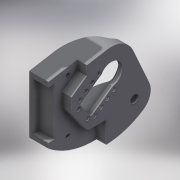
# Autodesk Inventor part: Arm - right shoulder v3
Saved by Autodesk Inventor 2017 (Build 210142000, 142)
## iProperties
Created: 2016-08-10
Part Number: Arm - right shoulder v3
Material: Generic
Document SubType Name: Modeling
Designer: Ali
Density: 1 g/cm^3
Appearance: Default
Author: Ali
Autodesk Inventor part; units mm, degrees
ref_plane "YZ Plane" through (0, 0, 0) normal (1, 0, 0) x (0, 1, 0)
ref_plane "XZ Plane" through (0, 0, 0) normal (0, 1, 0) x (-1, 0, 0)
ref_plane "XY Plane" through (0, 0, 0) normal (0, 0, 1) x (1, 0, 0)
sketch "Sketch1" plane through (0, 0, 0) normal (1, 0, 0) x (0, 1, 0)
  line L0 (0, 30) -> (51.1353, 38.6498)
  line L1 (78.1197, 24.2221) -> (94.819, -13.049)
  line L2 (0, -30) -> (0, 30)
  arc A0 (78.1197, 24.2221) -> (51.1353, 38.6498) centre (55.305, 14) ccw
  arc A1 (88.6362, -34.2101) -> (94.819, -13.049) centre (79.305, -20) ccw
  arc A2 (0, -30) -> (88.6362, -34.2101) centre (47.2144, 28.8695) ccw
  point P0 (0, 0)
  dimension "d14" = 55.305
  dimension "d15" = 14
  dimension "d16" = 17
  dimension "d17" = 34
  dimension "d18" = 24
  dimension "d19" = 25
  dimension "d25" = 60
  dimension "d26" = 30
  constraints: 7 end point, 6 point on circle, 4 tangent, 3 centre point, 1 midpoint, 1 vertical
  measures "d14" horizontal distance of point (0, 0) A0.centre
  measures "d15" vertical distance of point (0, 0) A0.centre
  measures "d16" radius of A1
  measures "d17" vertical distance of A1.centre A0.centre
  measures "d18" horizontal distance of A1.centre A0.centre
  measures "d19" radius of A0
  measures "d25" distance of L2.start L0.start
  measures "d26" distance of L0.start point (0, 0)
extrude "Extrusion1" add sketch "Sketch1" along normal blind 30
sketch "Sketch2" plane through (30, 0, 0) normal (1, 0, 0) x (0, 0, -1)
  circle A0 centre (-14, 55.305) radius 11.4
  arc A1 (-24.2221, 78.1197) -> (-38.6498, 51.1353) centre (-14, 55.305) ccw projected
  line L0 (-14, 55.305) -> (7.0104, 55.305) construction
  line L1 (-14, 55.305) -> (-0.1357, 35.6656) construction
  line L2 (-22.3737, 49.3936) -> (-3.342, 22.4345)
  line L3 (-3.342, 22.4345) -> (5.0317, 28.3459)
  line L4 (13.4054, 34.2572) -> (-5.6263, 61.2164)
  line L5 (-5.6263, 61.2164) -> (-22.3737, 49.3936)
  line L6 (5.0317, 28.3459) -> (13.4054, 34.2572)
  point P0 (0, 0)
  dimension "d6" = 22.8
  dimension "d8" = 54.78
  dimension "d9" = 20.5
  dimension "d10" = 33
  constraints: 14 end point, 6 perpendicular, 1 centre point, 1 coincident, 1 collinear, 1 horizontal, 1 midpoint, 1 point on line
  measures "d6" diameter of A0
  measures "d8" angle of L1 L0
  measures "d9" distance between parallel lines of L4 L2
  measures "d10" distance between parallel lines of L5 L3
extrude "Extrusion2" cut sketch "Sketch2" against normal through all
sketch "Sketch3" plane through (0, 0, 0) normal (-1, 0, 0) x (0, 0, 1)
  line L0 (19.496, 45.3173) -> (3.342, 22.4345) projected
  line L1 (3.342, 22.4345) -> (-13.4054, 34.2572) projected
  line L2 (-13.4054, 34.2572) -> (2.7487, 57.14) projected
  arc A0 (19.496, 45.3173) -> (2.7487, 57.14) centre (14, 55.305) ccw projected
  line L3 (30, 0) -> (38.6498, 51.1353) projected
  arc A1 (38.6498, 51.1353) -> (24.2221, 78.1197) centre (14, 55.305) ccw projected
  line L4 (24.2221, 78.1197) -> (-13.049, 94.819) projected
  arc A2 (-13.049, 94.819) -> (-34.2101, 88.6362) centre (-20, 79.305) ccw projected
  line L5 (-30, 0) -> (30, 0) projected
  line L6 (0.7237, 65.6142) -> (-22.5217, 32.6862)
  line L7 (2.7487, 57.14) -> (-13.4054, 34.2572) projected
  line L8 (-22.5217, 32.6862) -> (4.9137, 13.3183)
  line L9 (4.9137, 13.3183) -> (27.7177, 45.621)
  arc A3 (-2.0441, 50.3509) -> (14.7033, 38.5282) centre (14, 55.305) ccw construction
  arc A4 (0.2823, 64.989) -> (-2.0441, 50.3509) centre (14, 55.305) ccw construction
  arc A5 (27.7177, 45.621) -> (0.2823, 64.989) centre (14, 55.305) ccw
  arc A6 (14.7033, 38.5282) -> (27.7177, 45.621) centre (14, 55.305) ccw construction
  arc A7 (-34.2101, 88.6362) -> (-30, 0) centre (28.8695, 47.2144) ccw projected
  point P0 (0, 0)
  dimension "d20" = 33.583
  dimension "d21" = 16.7915
  dimension "d22" = 39.541
  constraints: 8 point on circle, 6 end point, 4 centre point, 3 point on line, 2 parallel, 2 tangent, 1 coincident, 1 perpendicular
  measures "d20" distance of L6.end L8.end
  measures "d21" distance from line of A0.centre L9
  measures "d22" distance from line of L8 A0.centre
extrude "Extrusion3" cut sketch "Sketch3" against normal blind 26 contours A5 L9 L8 L6
sketch "Sketch4" plane through (0, 0, 0) normal (-1, 0, 0) x (0, 0, 1)
  arc A0 (-13.049, 94.819) -> (-34.2101, 88.6362) centre (-20, 79.305) ccw projected
  arc A1 (-20, 62.305) -> (-3.8668, 84.6641) centre (-20, 79.305) ccw
  line L0 (-20, 62.305) -> (-49.8582, 62.305)
  line L1 (-49.8582, 62.305) -> (-49.8582, 92.5555)
  line L2 (-49.8582, 92.5555) -> (-2.7738, 107.9881)
  arc A2 (-3.8668, 84.6641) -> (-20, 62.305) centre (-20, 79.305) ccw construction
  line L3 (-20, 79.305) -> (-20, 114.7318) construction
  line L4 (2.7487, 57.14) -> (-13.4054, 34.2572) projected
  line L5 (-13.4054, 34.2572) -> (3.342, 22.4345) projected
  arc A3 (19.496, 45.3173) -> (2.7487, 57.14) centre (14, 55.305) ccw projected
  line L6 (-13.049, 94.819) -> (24.2221, 78.1197) projected
  line L7 (24.2221, 78.1197) -> (18.4359, 107.9881)
  line L8 (18.4359, 107.9881) -> (-2.7738, 107.9881)
  line L9 (24.2221, 78.1197) -> (-13.049, 94.819) projected
  arc A4 (0.6004, 88.7034) -> (-3.8668, 84.6641) centre (-0.7447, 85.7011) ccw
  point P0 (0, 0)
  dimension "d29" = 17
  constraints: 12 end point, 7 point on circle, 3 centre point, 3 tangent, 2 horizontal, 1 coincident, 1 perpendicular, 1 point on line, 1 vertical
  measures "d29" radius of A2
extrude "Extrusion4" cut sketch "Sketch4" against normal blind 24
sketch "Sketch5" plane through (0, 0, 0) normal (0, 0, 1) x (1, 0, 0)
  arc A0 (21, 63.7233) -> (0, 26.742) centre (43.0624, 26.742) ccw
  line L0 (0, 26.742) -> (0, 0)
  line L1 (34.277, 106.8627) -> (34.277, 0)
  line L2 (34.277, 0) -> (0, 0)
  line L3 (24, 94.819) -> (24, 88.7034) projected
  line L4 (21, 106.8627) -> (21, 63.7233)
  line L5 (21, 106.8627) -> (34.277, 106.8627)
  point P0 (24, 78.1197)
  dimension "d81" = 3
  constraints: 10 end point, 3 vertical, 2 point on circle, 1 centre point, 1 coincident, 1 horizontal, 1 perpendicular, 1 tangent
  measures "d81" distance between parallel lines of L3 L4
extrude "Extrusion5" cut sketch "Sketch5" along normal through all both and the other way through all keep common part
sketch "Sketch6" plane through (30, 0, 0) normal (1, 0, 0) x (0, 0, -1)
  line L0 (-3.342, 22.4345) -> (-19.496, 45.3173) projected
  arc A0 (-2.7487, 57.14) -> (-19.496, 45.3173) centre (-14, 55.305) ccw projected
  line L1 (-2.7487, 57.14) -> (13.4054, 34.2572) projected
  line L2 (13.4054, 34.2572) -> (-3.342, 22.4345) projected
  line L3 (-38.6498, 51.1353) -> (-30, 0) projected
  line L4 (-30, 0) -> (30, 0) projected
  arc A1 (30, 0) -> (34.2101, 88.6362) centre (-28.8695, 47.2144) ccw projected
  arc A2 (34.2101, 88.6362) -> (13.049, 94.819) centre (20, 79.305) ccw projected
  line L5 (13.049, 94.819) -> (-24.2221, 78.1197) projected
  arc A3 (-24.2221, 78.1197) -> (-38.6498, 51.1353) centre (-14, 55.305) ccw projected
  line L6 (-32.4314, 58.0054) -> (-4.2669, 18.1093) construction
  line L7 (-4.2669, 18.1093) -> (17.7906, 33.6807) construction
  line L8 (17.7906, 33.6807) -> (-7.019, 68.8244) construction
  line L9 (-3.342, 22.4345) -> (-19.496, 45.3173) projected
  line L10 (-2.7487, 57.14) -> (13.4054, 34.2572) projected
  line L11 (-21.2801, 42.2092) -> (-12.8111, 48.1878) construction
  line L12 (-14, 55.305) -> (-1.9064, 38.1739) construction
  point P0 (0, 0)
  point P1 (-16.6663, 35.6736)
  point P2 (-12.0526, 29.1381)
  point P3 (-7.4389, 22.6025)
  point P4 (0.7774, 57.7806)
  point P5 (5.3911, 51.245)
  point P6 (10.0049, 44.7095)
  point P7 (14.6186, 38.1739)
  point P8 (0.2263, 21.2813)
  point P9 (13.2974, 30.5088)
  dimension "d32" = 13.5
  dimension "d33" = 13.5
  dimension "d34" = 3
  dimension "d35" = 6.5
  dimension "d38" = 8
  dimension "d41" = 27
  dimension "d44" = 8
  constraints: 10 end point, 3 parallel, 3 perpendicular, 2 point on line, 1 symmetric about line, 9 other
  measures "d32" distance from line of A0.centre L6
  measures "d33" distance from line of L8 A0.centre
  measures "d34" distance between parallel lines of L7 L2
  measures "d35" distance from line of A0.centre L11
  measures "d38" distance of L11.start point (-16.666, 35.674)
  measures "d41" distance of L11.start point (0.777, 57.781)
  measures "d44" distance from line of point (0.226, 21.281) L12
hole "Hole1" at (30, 42.2092, 21.2801) at (30, 35.6736, 16.6663) at (30, 29.1381, 12.0526) at (30, 22.6025, 7.4389) at (30, 57.7806, -0.7774) at (30, 51.245, -5.3911) at (30, 44.7095, -10.0049) at (30, 38.1739, -14.6186) at (30, 21.2813, -0.2263) at (30, 30.5088, -13.2974) direction (-1, 0, 0) diameter 2.2 end through all counterbore diameter 4.2 counterbore depth 1.2
fillet "Fillet1" radius 2 2 edges at (28, 34.2572, -13.4054) (28, 22.4345, 3.342)
fillet "Fillet2" radius 8 2 edges at (13.2061, 32.6862, -22.5217) (13, 13.3183, 4.9137)
sketch "Sketch7" plane through (30, 0, 0) normal (1, 0, 0) x (0, 0, -1)
  circle A0 centre (0.2263, 21.2813) radius 2.1 projected
  circle A1 centre (10.0049, 44.7095) radius 2.1 projected
  circle A2 centre (0.7774, 57.7806) radius 2.1 projected
  circle A3 centre (-12.0526, 29.1381) radius 2.1 projected
  circle A4 centre (-21.2801, 42.2092) radius 2.1 projected
  circle A5 centre (-16.6663, 35.6736) radius 2.1 projected
  circle A6 centre (-7.4389, 22.6025) radius 2.1 projected
  circle A7 centre (5.3911, 51.245) radius 2.1 projected
  circle A8 centre (14.6186, 38.1739) radius 2.1 projected
  circle A9 centre (13.2974, 30.5088) radius 2.1 projected
  line L0 (-4.4954, 24.0684) -> (-19.496, 45.3173) projected
  arc A10 (-2.7487, 57.14) -> (-19.496, 45.3173) centre (-14, 55.305) ccw projected
  line L1 (-2.7487, 57.14) -> (12.2519, 35.8911) projected
  arc A11 (11.7715, 33.1038) -> (12.2519, 35.8911) centre (10.618, 34.7377) ccw projected
  line L2 (11.7715, 33.1038) -> (-1.7081, 23.5879) projected
  arc A12 (-4.4954, 24.0684) -> (-1.7081, 23.5879) centre (-2.8615, 25.2218) ccw projected
  line L3 (-38.6498, 51.1353) -> (-30, 0) projected
  line L4 (-30, 0) -> (30, 0) projected
  arc A13 (30, 0) -> (34.2101, 88.6362) centre (-28.8695, 47.2144) ccw projected
  arc A14 (34.2101, 88.6362) -> (13.049, 94.819) centre (20, 79.305) ccw projected
  line L5 (13.049, 94.819) -> (-24.2221, 78.1197) projected
  arc A15 (-24.2221, 78.1197) -> (-38.6498, 51.1353) centre (-14, 55.305) ccw projected
  line L6 (-38.6498, 51.1353) -> (-30, 0) projected
  line L7 (-25.2951, 30) -> (-14, 14)
  line L8 (0, 14) -> (24, 30.9427)
  line L9 (24, 50) -> (24, 30.9427)
  line L10 (24, 50) -> (46.543, 50)
  line L11 (-14, 14) -> (0, 14)
  line L12 (-35.0747, 30) -> (-25.2951, 30)
  line L13 (0, 14) -> (34.2101, 14) construction
  line L14 (0, 0) -> (0, 14) construction
  dimension "d56" = 14
  dimension "d57" = 24
  dimension "d58" = 50
  dimension "d59" = 30
  dimension "d60" = 14
  dimension "d74" = 25.2951
  dimension "d75" = 35.22
  dimension "d76" = 125.22
  constraints: 16 end point, 4 horizontal, 2 vertical, 1 parallel, 1 perpendicular, 1 point on circle, 1 point on line
  measures "d56" distance between parallel lines of L4 L11
  measures "d57" distance from line of L9 L14.start
  measures "d58" distance between parallel lines of L10 L4
  measures "d59" distance between parallel lines of L4 L12
  measures "d60" distance of L7.end L8.start
  measures "d74" horizontal distance of L7.start L14.start
  measures "d75" angle of L13 L8
  measures "d76" angle of L7 L13
extrude "Extrusion6" cut sketch "Sketch7" against normal blind 10 contours L12 L7 L11 L8 L9 L10 A13 L4 L3
sketch "Sketch8" plane through (0, 0, 0) normal (-1, 0, 0) x (0, 0, 1)
  line L0 (-30, 0) -> (30, 0) projected
  arc A0 (-46.543, 50) -> (-30, 0) centre (28.8695, 47.2144) ccw projected
  line L1 (-24, 50) -> (-46.543, 50) projected
  line L2 (-24, 30.9427) -> (-24, 50) projected
  line L3 (0, 14) -> (-24, 30.9427) projected
  line L4 (14, 14) -> (0, 14) projected
  line L5 (25.2951, 30) -> (14, 14) projected
  line L6 (35.0747, 30) -> (25.2951, 30) projected
  line L7 (30, 0) -> (35.0747, 30) projected
  line L8 (-29, 20) -> (26, 20) construction
  point P0 (0, 0)
  point P1 (-34, 40)
  dimension "d62" = 20
  dimension "d63" = 5
  dimension "d64" = 55
  dimension "d65" = 26
  dimension "d66" = 20
  constraints: 2 end point, 1 horizontal
  measures "d62" vertical distance of L8.start point (-34, 40)
  measures "d63" horizontal distance of point (-34, 40) L8.start
  measures "d64" distance of L8.end L8.start
  measures "d65" horizontal distance of L8.end point (0, 0)
  measures "d66" distance from line of point (0, 0) L8
hole "Hole2" at (0, 40, -34) at (0, 20, -29) at (0, 20, 26) direction (1, 0, 0) diameter 4.2 end through all counterbore diameter 7.2 counterbore depth 10
sketch "Sketch9" plane through (0, 0, -30) normal (0, -1, 0) x (1, 0, 0)
  line L0 (20, 0) -> (20, 60) projected
  line L1 (20, 5) -> (4, 5)
  line L2 (4, 5) -> (4, 55)
  line L3 (4, 55) -> (20, 55)
  line L4 (20, 55) -> (20, 5)
  point P0 (0, 30)
  dimension "d77" = 50
  dimension "d78" = 16
  dimension "d101" = 25
  constraints: 8 end point, 2 parallel, 1 horizontal, 1 perpendicular, 1 point on line
  measures "d77" distance of L1.end L2.end
  measures "d78" distance of L1.start L1.end
  measures "d101" distance from line of point (0, 30) L1
extrude "Extrusion7" cut sketch "Sketch9" against normal blind 6
fillet "Fillet3" radius 4.75 2 edges at (21, 63.7233, -6.9066) (21, 63.7233, 33.0344)
sketch "Sketch10" plane through (24, 0, 0) normal (-1, 0, 0) x (0, 0, 1)
  arc A0 (-13.049, 94.819) -> (-34.2101, 88.6362) centre (-20, 79.305) ccw projected
  circle A1 centre (-20, 79.305) radius 6
  point P0 (0, 0)
  dimension "d83" = 12
  constraints: 1 centre point, 1 coincident
  measures "d83" diameter of A1
extrude "Extrusion8" add sketch "Sketch10" along normal blind 1
sketch "Sketch11" plane through (23, 79.305, -20) normal (-1, 0, 0) x (0, 0, 1)
  circle A0 centre (0, 0) radius 6 projected
  circle A1 centre (0, 0) radius 4
  point P0 (20, -79.305)
  dimension "d86" = 8
  constraints: 1 centre point, 1 coincident
  measures "d86" diameter of A1
extrude "Extrusion9" add sketch "Sketch11" along normal blind 7 contours A1
hole "Hole3" at (30, 79.305, -20) direction (-1, 0, 0) diameter 4.2 end through all counterbore diameter 8 counterbore depth 4
chamfer "Chamfer1" distance 0.5 angle 45 1 edges at (16, 79.305, -24)
equation "\"d26\" = 0.5 * d25"
equation "\"d21\" = 0.5 * d20"
equation "\"d33\" = d32"
body "Solid1"
